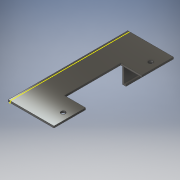
# Autodesk Inventor part: side
Saved by Autodesk Inventor 2016 (Build 200138000, 138)
## iProperties
Created: 2015-10-31
Part Number: side
Material: Generic
Document SubType Name: Modeling
Designer: rossmosier
Density: 1 g/cm^3
Appearance: Chrome - Polished
Author: rossmosier
Autodesk Inventor part; units mm, degrees
ref_plane "YZ Plane" through (0, 0, 0) normal (1, 0, 0) x (0, 1, 0)
ref_plane "XZ Plane" through (0, 0, 0) normal (0, 1, 0) x (-1, 0, 0)
ref_plane "XY Plane" through (0, 0, 0) normal (0, 0, 1) x (1, 0, 0)
sketch "Sketch1" plane through (0, 0, 0) normal (0, 1, 0) x (-1, 0, 0)
  line L0 (0, 0) -> (-88.9, 0)
  line L1 (-88.9, -114.3) -> (-88.9, -317.5)
  line L2 (-88.9, -431.8) -> (0, -431.8)
  line L3 (0, -431.8) -> (0, 0)
  line L4 (-88.9, 0) -> (-165.1, 0)
  line L5 (-165.1, 0) -> (-165.1, -114.3)
  line L6 (-165.1, -114.3) -> (-88.9, -114.3)
  line L7 (-88.9, -114.3) -> (-88.9, 0)
  line L8 (-88.9, -431.8) -> (-165.1, -431.8)
  line L9 (-165.1, -431.8) -> (-165.1, -317.5)
  line L10 (-165.1, -317.5) -> (-88.9, -317.5)
  line L11 (-88.9, -317.5) -> (-88.9, -431.8)
  line L12 (-88.9, -374.65) -> (-139.7, -374.65) construction
  line L13 (-88.9, -58.8342) -> (-139.7, -58.8342) construction
  circle A0 centre (-139.7, -58.8342) radius 7.9375
  circle A1 centre (-139.7, -374.65) radius 7.9375
  dimension "d0" = 88.9
  dimension "d1" = 431.8
  dimension "d2" = 76.2
  dimension "d3" = 114.3
  dimension "d4" = 76.2
  dimension "d5" = 114.3
  dimension "d6" = 50.8
  dimension "d7" = 15.875
  dimension "d8" = 15.875
  constraints: 28 end point, 6 parallel, 5 horizontal, 3 perpendicular, 2 centre point, 2 coincident, 1 midpoint, 1 point on line
  measures "d0" distance of L2.end L2.start
  measures "d1" distance of L2.start L0.end
  measures "d2" distance of L1.start L5.end
  measures "d3" distance of L5.end L4.end
  measures "d4" distance of L1.end L9.end
  measures "d5" distance of L8.end L9.end
  measures "d6" distance of L12.start L12.end
  measures "d7" diameter of A0
  measures "d8" diameter of A1
extrude "Extrusion1" add sketch "Sketch1" along normal blind 6.35
sketch "Sketch2" plane through (0, 0, 0) normal (0, -1, 0) x (1, 0, 0)
  circle A0 centre (139.7, -58.8342) radius 7.9375 projected
  circle A1 centre (139.7, -374.65) radius 7.9375 projected
  line L0 (165.1, -431.8) -> (0, -431.8) projected
  line L1 (165.1, -317.5) -> (165.1, -431.8) projected
  line L2 (88.9, -317.5) -> (165.1, -317.5) projected
  line L3 (88.9, -114.3) -> (88.9, -317.5) projected
  line L4 (165.1, -114.3) -> (88.9, -114.3) projected
  line L5 (165.1, 0) -> (165.1, -114.3) projected
  line L6 (0, 0) -> (165.1, 0) projected
  line L7 (0, -431.8) -> (0, 0) projected
  line L8 (0, -431.8) -> (0, 0) projected
  line L9 (0, -431.8) -> (6.35, -431.8)
  line L10 (6.35, -431.8) -> (6.35, -330.2)
  line L11 (6.35, -330.2) -> (0, -330.2)
  line L12 (0, -330.2) -> (0, -431.8)
  line L13 (88.9, -431.8) -> (82.55, -431.8)
  line L14 (82.55, -431.8) -> (82.55, -330.2)
  line L15 (82.55, -330.2) -> (88.9, -330.2)
  line L16 (88.9, -330.2) -> (88.9, -431.8)
  dimension "d11" = 6.35
  dimension "d12" = 101.6
  constraints: 16 end point, 4 parallel, 2 horizontal, 2 perpendicular, 2 point on line
  measures "d11" distance of L11.end L10.end
  measures "d12" distance of L10.end L9.end
extrude "Extrusion2" add sketch "Sketch2" along normal blind 69.85 contours L0 L14 L15 L16 | L0 L7 L11 L10
sketch "Sketch3" plane through (0, 6.35, -431.8) normal (-1, 0, 0) x (0, 0, 1)
  line L0 (101.6, -6.35) -> (431.8, -6.35) projected
  line L1 (431.8, -6.35) -> (431.8, 0) projected
  line L2 (0, 0) -> (431.8, 0) projected
  line L3 (0, -76.2) -> (0, 0) projected
  line L4 (101.6, -76.2) -> (0, -76.2) projected
  line L5 (101.6, -6.35) -> (101.6, -76.2) projected
  line L6 (101.6, -6.35) -> (101.6, -76.2) projected
  line L7 (0, -76.2) -> (101.6, -76.2)
  line L8 (101.6, -76.2) -> (101.6, -69.85)
  line L9 (101.6, -69.85) -> (0, -69.85)
  line L10 (0, -69.85) -> (0, -76.2)
  dimension "d15" = 6.35
  constraints: 8 end point, 2 parallel, 1 horizontal, 1 perpendicular, 1 point on line
  measures "d15" distance of L8.end L7.end
sketch "Sketch4" plane through (88.9, 0, -330.2) normal (1, 0, 0) x (0, 0, -1)
  line L0 (0, 0) -> (101.6, 0) projected
  line L1 (0, 0) -> (0, -69.85) projected
  line L2 (101.6, -69.85) -> (0, -69.85) projected
  line L3 (101.6, 0) -> (101.6, -69.85) projected
  line L4 (0, 0) -> (0, -69.85) projected
  line L5 (101.6, -69.85) -> (0, -69.85)
  line L6 (0, -69.85) -> (0, -63.4998)
  line L7 (0, -63.4998) -> (101.6, -63.4998)
  line L8 (101.6, -63.4998) -> (101.6, -69.85)
  point P0 (-330.2, 0)
  constraints: 8 end point, 2 parallel, 1 horizontal, 1 perpendicular, 1 point on line
extrude "Extrusion3" add sketch "Sketch3" along normal blind 6.35 contours L5 L4 L3 L9
extrude "Extrusion4" add sketch "Sketch4" along normal blind 6.35 contours L7 L3 L2 L1
sketch "Sketch5" plane through (6.35, 0, -330.2) normal (1, 0, 0) x (0, 0, -1)
  line L0 (101.6, -63.5) -> (0, -63.5) projected
  line L1 (0, 0) -> (0, -63.5) projected
  line L2 (0, 0) -> (-330.2, 0) projected
  line L3 (-330.2, 0) -> (-330.2, 6.35) projected
  line L4 (101.6, 6.35) -> (-330.2, 6.35) projected
  line L5 (101.6, -63.5) -> (101.6, 6.35) projected
  point P0 (50.8, -28.575)
body "Solid1"
